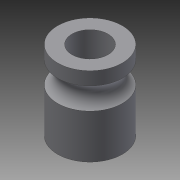
# Autodesk Inventor part: MK8_Drive_Gear
Saved by Autodesk Inventor 2014 SP2 (Build 180246200, 246)
## iProperties
Created: 2014-09-30
Part Number: MK8_Drive_Gear
Material: Generic
Document SubType Name: Modeling
Designer: ThatOtherGuy
Density: 1 g/cm^3
Appearance: Default
Author: ThatOtherGuy
Autodesk Inventor part; units mm, degrees
ref_plane "YZ Plane" through (0, 0, 0) normal (1, 0, 0) x (0, 1, 0)
ref_plane "XZ Plane" through (0, 0, 0) normal (0, 1, 0) x (-1, 0, 0)
ref_plane "XY Plane" through (0, 0, 0) normal (0, 0, 1) x (1, 0, 0)
sketch "Sketch1" plane through (0, 0, 0) normal (0, 0, 1) x (1, 0, 0)
  circle A0 centre (0, 0) radius 4.5
  circle A1 centre (0, 0) radius 2.5
  dimension "d0" = 9
  dimension "d1" = 5
  constraints: 2 centre point, 2 coincident
  measures "d0" diameter of A0
  measures "d1" diameter of A1
extrude "Extrusion1" add sketch "Sketch1" along normal blind 11
sketch "Sketch2" plane through (0, 0, 0) normal (1, 0, 0) x (0, 1, 0)
  circle A0 centre (5.15, 7.65) radius 1.65
  line L0 (-4.5, 0) -> (4.5, 0) projected
  line L1 (0, 0) -> (0, 16.0894)
  dimension "d7" = 7.65
  dimension "d8" = 5.15
  dimension "d9" = 3.3
  constraints: 2 end point, 1 centre point, 1 perpendicular
  measures "d7" distance from line of L0 A0.centre
  measures "d8" horizontal distance of L1.start A0.centre
  measures "d9" diameter of A0
revolve "Revolution1" cut sketch "Sketch2" angle 360 about axis through (0, 0, 0) along (0, 0, 1)
sketch "Sketch3" plane through (0, 0, 0) normal (1, 0, 0) x (0, 1, 0)
  circle A0 centre (0, 3.1) radius 1.25
  point P0 (0, 0)
  dimension "d11" = 2.5
  dimension "d12" = 3.1
  constraints: 1 centre point, 1 vertical alignment
  measures "d11" diameter of A0
  measures "d12" distance of point (0, 0) A0.centre
extrude "Extrusion2" cut sketch "Sketch3" against normal blind 11
thread "Thread1" size "M2.5x0.45" class "6H" standard "ANSI Metric M Profile" full length
body "Solid1"
